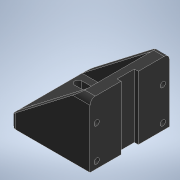
# Autodesk Inventor part: 26_Laser_carriage_V2
Saved by Autodesk Inventor 2022.2 (Build 262287010, 287A)
## iProperties
Created: 2022-05-02
Part Number: 26_Laser_carriage_V2
Material: PET-Kunststoff
Document SubType Name: Modeling
Designer: MXBD
Density: 1.541 g/cm^3
Appearance: Gummi - Schwarz
Author: MXBD
Autodesk Inventor part; units mm, degrees
ref_plane "YZ Plane" through (0, 0, 0) normal (1, 0, 0) x (0, 1, 0)
ref_plane "XZ Plane" through (0, 0, 0) normal (0, 1, 0) x (-1, 0, 0)
ref_plane "XY Plane" through (0, 0, 0) normal (0, 0, 1) x (1, 0, 0)
sketch "Skizze1" plane through (0, 0, 0) normal (0, 1, 0) x (-1, 0, 0)
  line L0 (-30, 30) -> (30, 30)
  line L1 (30, 30) -> (30, -30)
  line L2 (30, -30) -> (-30, -30)
  line L3 (-30, -30) -> (-30, 30)
  line L4 (-30, 30) -> (30, -30) construction
  line L5 (30, 30) -> (-30, -30) construction
  point P0 (0, 0)
  dimension "d0" = 60
  dimension "d1" = 60
  constraints: 12 end point, 2 midpoint, 2 parallel, 1 horizontal, 1 perpendicular
  measures "d0" distance of L1.end L2.end
  measures "d1" distance of L0.end L1.end
extrude "Extrusion1" add sketch "Skizze1" along normal blind 8
sketch "Skizze2" plane through (0, 8, 0) normal (0, 1, 0) x (1, 0, 0)
  line L0 (-30, -30) -> (30, -30) projected
  line L1 (30, 30) -> (-30, 30) projected
  line L2 (30, -30) -> (22, -30)
  line L3 (22, -30) -> (22, 30)
  line L4 (22, 30) -> (30, 30)
  line L5 (30, 30) -> (30, -30)
  point P0 (0, 0)
  dimension "d4" = 8
  constraints: 8 end point, 2 parallel, 1 horizontal, 1 perpendicular, 1 point on line
  measures "d4" distance of L3.end L4.end
extrude "Extrusion2" add sketch "Skizze2" along normal blind 40
sketch "Skizze3" plane through (0, 8, 0) normal (0, 1, 0) x (1, 0, 0)
  line L0 (42, 0) -> (-42, 0) projected
  line L1 (22, 30) -> (22, -30) projected
  point P0 (0, 0)
  point P1 (18, -12.5)
  point P2 (18, 12.5)
  point P3 (-7, 12.5)
  point P4 (-7, -12.5)
  dimension "d7" = 25
  dimension "d8" = 25
  dimension "d9" = 4
  constraints: 2 symmetric about line, 1 horizontal alignment
  measures "d7" distance of point (18, 12.5) point (18, -12.5)
  measures "d8" distance of point (-7, 12.5) point (18, 12.5)
  measures "d9" distance from line of point (18, -12.5) L1
hole "Bohrung1" at (18, 8, 12.5) at (18, 8, -12.5) at (-7, 8, -12.5) at (-7, 8, 12.5) direction (0, -1, 0) diameter 3.4 end through all counterbore diameter 6.5 counterbore depth 3.4 clearance for "Inbusschraube ISO 4762" size "M3" standard "ISO"
sketch "Skizze4" plane through (30, 0, 30) normal (1, 0, 0) x (0, 0, -1)
  line L0 (30, -9.6) -> (30, 57.6) projected
  circle A0 centre (5, 5) radius 2
  circle A1 centre (55, 5) radius 2
  line L1 (0, 48) -> (60, 48) projected
  line L2 (0, 0) -> (60, 0) projected
  circle A2 centre (55, 30) radius 2
  circle A3 centre (5, 30) radius 2
  point P0 (30, 0)
  dimension "d17" = 4
  dimension "d18" = 50
  dimension "d22" = 5
  dimension "d25" = 25
  constraints: 4 centre point, 3 equal radius, 1 vertical alignment, 2 other
  measures "d17" diameter of A0
  measures "d18" distance of A1.centre A0.centre
  measures "d22" distance from line of A0.centre L2
  measures "d25" distance of A1.centre A2.centre
extrude "Extrusion3" cut sketch "Skizze4" against normal blind 7
sketch "Skizze5" plane through (0, 0, 0) normal (0, 0, 1) x (1, 0, 0)
  line L0 (30, 48) -> (22, 48) projected
  line L1 (-30, 0) -> (-30, 8) projected
  line L2 (22, 48) -> (-30, 8)
  line L3 (-30, 8) -> (22, 8)
  line L4 (22, 8) -> (22, 48)
  point P0 (0, 0)
  constraints: 6 end point, 2 perpendicular
extrude "Extrusion4" add sketch "Skizze5" against normal blind 6 from surface at 30
mirror "Spiegeln1" about plane through (0, 0, 0) normal (0, 0, 1) of "Extrusion4"
sketch "Skizze6" plane through (0, 48, 0) normal (0, 1, 0) x (1, 0, 0)
  line L0 (33, -6.5) -> (27, -6.5)
  line L1 (27, -6.5) -> (27, 6.5)
  line L2 (27, 6.5) -> (33, 6.5)
  line L3 (33, 6.5) -> (33, -6.5)
  line L4 (30, -30) -> (30, 30) projected
  line L5 (33, -6.5) -> (27, 6.5) construction
  line L6 (27, -6.5) -> (33, 6.5) construction
  point P0 (0, 0)
  point P1 (30, 0)
  point P2 (30, -6.5)
  point P3 (30, 6.5)
  dimension "d26" = 3
  dimension "d27" = 13
  constraints: 12 end point, 3 midpoint, 2 parallel, 1 horizontal, 1 perpendicular
  measures "d26" distance between parallel lines of L4 L1
  measures "d27" distance between parallel lines of L0 L2
extrude "Extrusion5" cut sketch "Skizze6" against normal through all contours L0 L1 L2 L4
sketch "Skizze7" plane through (0, 8, 0) normal (0, 1, 0) x (1, 0, 0)
  line L0 (-25, 16.1375) -> (-16, 16.1375) construction
  line L1 (-25, 13.3875) -> (-16, 13.3875)
  line L2 (-16, 18.8875) -> (-25, 18.8875)
  arc A0 (-25, 18.8875) -> (-25, 13.3875) centre (-25, 16.1375) ccw
  arc A1 (-16, 13.3875) -> (-16, 18.8875) centre (-16, 16.1375) ccw
  line L3 (-30, 24) -> (-30, -24) projected
  point P0 (0, 0)
  point P1 (-20.5, 16.1375)
  dimension "d30" = 5.5
  dimension "d31" = 9
  dimension "d32" = 9.5
  constraints: 8 end point, 4 point on circle, 4 tangent, 2 centre point, 1 horizontal, 1 midpoint, 1 parallel
  measures "d30" distance between parallel lines of L1 L2
  measures "d31" distance of L0.end L0.start
  measures "d32" distance from line of point (-20.5, 16.138) L3
extrude "Extrusion6" cut sketch "Skizze7" against normal through all
mirror "Spiegeln2" about plane through (0, 0, 0) normal (0, 0, 1) of "Extrusion6"
fillet "Rundung1" radius 4 4 edges at (26, 48, 30) (26, 48, -30) (-30, 4, 30) (-30, 4, -30)
